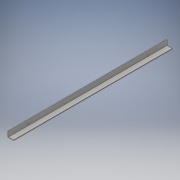
# Autodesk Inventor part: 27.5 L
Saved by Autodesk Inventor 2016 SP2 (Build 200236200, 236)
## iProperties
Created: 2018-01-20
Part Number: 27.5 L
Material: Generic
Document SubType Name: Modeling
Designer: CAD
Density: 1 g/cm^3
Appearance: Default
Author: CAD
Autodesk Inventor part; units mm, degrees
ref_plane "YZ Plane" through (0, 0, 0) normal (1, 0, 0) x (0, 1, 0)
ref_plane "XZ Plane" through (0, 0, 0) normal (0, 1, 0) x (-1, 0, 0)
ref_plane "XY Plane" through (0, 0, 0) normal (0, 0, 1) x (1, 0, 0)
sketch "Sketch1" plane through (0, 0, 0) normal (0, 0, 1) x (1, 0, 0)
  line L0 (0, 0) -> (-25.4, 0)
  line L1 (-25.4, 0) -> (-25.4, 25.4)
  line L2 (0, 3.175) -> (-22.225, 3.175)
  line L3 (-22.225, 3.175) -> (-22.225, 25.4)
  line L4 (0, 3.175) -> (0, 0)
  line L5 (-25.4, 25.4) -> (-22.225, 25.4)
  dimension "d0" = 25.4
  dimension "d1" = 25.4
  dimension "d2" = 3.175
  constraints: 12 end point, 2 horizontal, 2 perpendicular, 1 vertical, 1 other
  measures "d0" distance of L0.start L0.end
  measures "d1" distance of L0.end L1.end
  measures "d2" distance between parallel lines of L0 L2
extrude "Extrusion1" add sketch "Sketch1" along normal blind 698.5
sketch "Sketch2" plane through (-22.225, 3.175, 0) normal (1, 0, 0) x (0, 0, -1)
  line L0 (0, 22.225) -> (0, 0) projected
  line L1 (0, 11.1125) -> (0, 6.0325)
  line L2 (0, 6.0325) -> (-85.725, 6.0325)
  line L3 (0, 22.225) -> (-698.5, 22.225) projected
  line L4 (-349.25, 22.225) -> (-349.25, 11.1125)
  line L5 (-698.5, 22.225) -> (-698.5, 0)
  line L6 (-698.5, 11.1125) -> (-698.5, 6.0325)
  line L7 (-698.5, 6.0325) -> (-612.775, 6.0325)
  line L8 (-698.5, 22.225) -> (0, 22.225)
  point P0 (0, -3.175)
  point P1 (-698.5, -3.175)
  dimension "d5" = 5.08
  dimension "d6" = 85.725
  constraints: 14 end point, 7 symmetric about line, 2 coincident, 2 midpoint, 2 point on line, 1 perpendicular, 1 vertical
  measures "d5" distance of L1.start L1.end
  measures "d6" distance of L1.end L2.end
hole "Hole1" at (-22.225, 9.2075, 612.775) at (-22.225, 9.2075, 85.725) direction (-1, 0, 0) diameter 6.35 end through all
body "Solid1"
